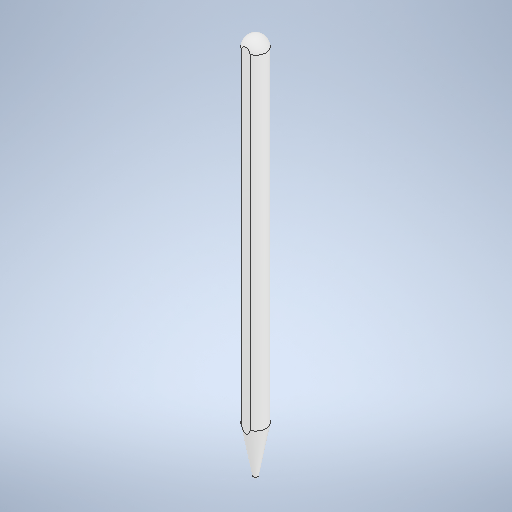
# Autodesk Inventor part: stylus_pen
Saved by Autodesk Inventor 2025.1 (Build 291241000, 241)
## iProperties
Created: 2024-08-22
Part Number: stylus_pen
Material: Acetal Resin, White
Document SubType Name: Modeling
Designer: pedro
Density: 1.425 g/cm^3
Appearance: Smooth - White
Author: pedro
Autodesk Inventor part; units mm, degrees
ref_plane "YZ Plane" through (0, 0, 0) normal (1, 0, 0) x (0, 1, 0)
ref_plane "XZ Plane" through (0, 0, 0) normal (0, 1, 0) x (-1, 0, 0)
ref_plane "XY Plane" through (0, 0, 0) normal (0, 0, 1) x (1, 0, 0)
sketch "Sketch1" plane through (0, 0, 0) normal (0, 1, 0) x (-1, 0, 0)
  arc A0 (1.8655, -4.15) -> (-1.8655, -4.15) centre (0, 0) ccw
  line L0 (1.8655, -4.15) -> (-1.8655, -4.15)
  dimension "d26" = 0.4
  dimension "d27" = 9.1
  constraints: 2 end point, 2 point on circle, 1 centre point, 1 horizontal
  measures "d26" distance edge to line of A0 L0
  measures "d27" diameter of A0
extrude "Extrusion1" add sketch "Sketch1" along normal blind 140
sketch "Sketch6" plane through (0, 0, 0) normal (0, 0, 1) x (1, 0, 0)
  line L0 (4.55, 140) -> (-4.55, 140) projected
  arc A0 (4.55, 140) -> (0, 144.55) centre (0, 140) ccw
  line L1 (0, 140) -> (0, 144.55)
  line L2 (0, 140) -> (4.55, 140)
  point P0 (0, 0)
  point P1 (-1.8655, 140)
  point P2 (1.8655, 140)
  constraints: 5 end point, 3 point on circle, 1 centre point, 1 collinear, 1 midpoint, 1 point on line, 1 vertical
revolve "Revolution4" add sketch "Sketch6" angle 360 about axis through (0, 140, 0) along (0, 1, 0)
thicken "Thicken7" operation cut thickness 2 both sides no extend neighbours no toward (0, 1, 0) faces at (0, 140, -4.2833)
sketch "Sketch7" plane through (0, 0, 0) normal (0, 0, 1) x (1, 0, 0)
  line L0 (-4.55, 0) -> (-4.55, 140) projected
  line L1 (-4.55, 0) -> (-1, -19.6824)
  line L2 (4.55, 0) -> (-4.55, 0) projected
  line L3 (1, -19.6824) -> (4.55, 0)
  line L4 (1.8655, 0) -> (-1.8655, 0) projected
  arc A0 (-1, -19.6824) -> (1, -19.6824) centre (0, -19.6824) ccw
  line L5 (4.55, 0) -> (0, 0)
  line L6 (0, -20.6824) -> (0, 0)
  point P0 (0, 0)
  dimension "d31" = 20
  dimension "d33" = 20
  constraints: 8 end point, 3 point on circle, 2 midpoint, 1 centre point, 1 collinear, 1 perpendicular, 1 point on line
  measures "d31" distance of L1.start L1.end
  measures "d33" distance of L3.start L2.start
revolve "Revolution5" add sketch "Sketch7" angle 360 about axis through (0, -20.6824, 0) along (0, 1, 0) contours L6 L2 L3 A0
thicken "Thicken8" operation cut thickness 3 both sides no extend neighbours no toward (0, -1, 0) faces at (-0.318, 0, -4.2496)
body "Solid1"
